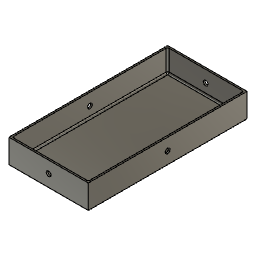
panel maker v4 (Autodesk Fusion 360 design; units mm, degrees)
Autodesk Fusion 360 part; units mm, degrees
sketch "Sketch2" plane through (0, 0, 0) normal (0, 1, 0) x (1, 0, 0)
  line L0 (0, 0) -> (50, 0)
  line L1 (50, 0) -> (50, -15)
  line L2 (50, -15) -> (0, -15)
  line L3 (0, -15) -> (0, 0)
  dimension "d15" = 50
  dimension "d16" = 15
  constraint horizontal L0
  constraint vertical L1
  constraint horizontal L2
  constraint vertical L3
  constraint coincident L0.start L3.end
  measures "d15" distance of L1.end L2.end
  measures "d16" distance of L0.start L2.end
extrude "Extrude1" add sketch "Sketch2" along normal blind 100
shell "Shell2" thickness 1 removed faces 1 at (33.3333, 33.3333, 15)
sketch "Sketch3" plane through (0, 0, 0) normal (0, -1, 0) x (1, 0, 0)
  line L0 (50, 15) -> (0, 15)
  line L1 (0, 15) -> (0, 0)
  line L2 (0, 0) -> (50, 0)
  line L3 (50, 0) -> (50, 15)
  circle A0 centre (25, 7.5) radius 1.5
  dimension "d20" = 3
  dimension "d21" = 25
  dimension "d22" = 7.5
  measures "d20" diameter of A0
  measures "d21" distance of L1 A0.centre
  measures "d22" distance of L0 A0.centre
extrude "Extrude2" cut sketch "Sketch3" against normal blind 100 contours A0
sketch "Sketch4" plane through (50, 0, 0) normal (1, 0, 0) x (0, 1, 0)
  line L0 (0, 15) -> (0, 0)
  line L1 (0, 0) -> (100, 0)
  line L2 (100, 0) -> (100, 15)
  line L3 (100, 15) -> (0, 15)
  circle A0 centre (50, 7.5) radius 1.5
  dimension "d25" = 3
  dimension "d26" = 50
  dimension "d27" = 7.5
  measures "d25" diameter of A0
  measures "d26" distance of L0 A0.centre
  measures "d27" distance of L3 A0.centre
extrude "Extrude3" cut sketch "Sketch4" against normal blind 50 contours A0
fillet "Fillet1" radius 1 3 edges at (1, 99, 8) (1, 50, 1) (25, 99, 1)
fillet "Fillet2" radius 1 3 edges at (1, 1, 8.5) (1.2929, 1, 1.2929) (25.5, 1, 1)
fillet "Fillet3" radius 1 5 edges at (49, 99, 8.5) (49, 98.7071, 1.2929) (49, 50, 1) (49, 1.2929, 1.2929) (49, 1, 8.5)
equation "Length = 100 mm"
equation "Width = 50 mm"
equation "Height = 15 mm"
equation "Wall = 1 mm"
equation "LPos = Length / 2"
equation "WPos = Width / 2"
equation "HPos = Height / 2"
equation "Screw = 3 mm"
equation "d15 = Width"
equation "d16 = Height"
equation "d17 = Length"
equation "d19 = Wall"
equation "d20 = Screw"
equation "d21 = WPos"
equation "d22 = HPos"
equation "d23 = -Length"
equation "d25 = Screw"
equation "d26 = LPos"
equation "d27 = HPos"
equation "d28 = -Width"
equation "Internal_fillet = 1 mm"
equation "d32 = Internal_fillet"
equation "d34 = Internal_fillet"
equation "d36 = Internal_fillet"
